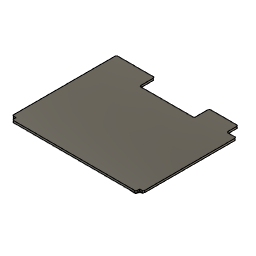
HexDeck_Printed_v0.1 (Autodesk Fusion 360 design; units mm, degrees)
Autodesk Fusion 360 part; units mm, degrees
(part 1 of 2)
sketch "Sketch1" plane through (0, 0, 86) normal (0, 0, 1) x (-1, 0, 0)
  line L0 (-104.5, -11) -> (-104.5, -155)
  arc A0 (-104.5, -155) -> (-102.5, -157) centre (-102.5, -155) ccw
  line L1 (-102.5, -157) -> (-91.5, -157)
  arc A1 (-89.5, -159) -> (-91.5, -157) centre (-91.5, -159) ccw
  line L2 (-89.5, -159) -> (-89.5, -173)
  arc A2 (-89.5, -173) -> (-87.5, -175) centre (-87.5, -173) ccw
  line L3 (-87.5, -175) -> (-45.5, -175)
  arc A3 (-45.5, -175) -> (-43.5, -173) centre (-45.5, -173) ccw
  line L4 (-43.5, -173) -> (-43.5, -153)
  arc A4 (-41.5, -151) -> (-43.5, -153) centre (-41.5, -153) ccw
  line L5 (-41.5, -151) -> (41.5, -151)
  arc A5 (43.5, -153) -> (41.5, -151) centre (41.5, -153) ccw
  line L6 (43.5, -153) -> (43.5, -173)
  arc A6 (43.5, -173) -> (45.5, -175) centre (45.5, -173) ccw
  arc A7 (98.5, -8.5) -> (99, -9) centre (99, -8.5) ccw
  line L7 (98.5, -8.5) -> (98.5, -5)
  arc A8 (98.5, -5) -> (96.5, -3) centre (96.5, -5) ccw
  line L8 (96.5, -3) -> (-96.5, -3)
  arc A9 (-96.5, -3) -> (-98.5, -5) centre (-96.5, -5) ccw
  line L9 (-98.5, -5) -> (-98.5, -8.5)
  arc A10 (-99, -9) -> (-98.5, -8.5) centre (-99, -8.5) ccw
  line L10 (-99, -9) -> (-102.5, -9)
  arc A11 (-102.5, -9) -> (-104.5, -11) centre (-102.5, -11) ccw
  circle A12 centre (-6, -134.5) radius 1.75
  circle A13 centre (-91, -12) radius 1.75
  circle A14 centre (85.1504, -110.8568) radius 1.7
  circle A15 centre (20.415, -94.6658) radius 1.7
  circle A16 centre (57.915, -46.1658) radius 1.7
  circle A17 centre (20.415, -32.4658) radius 1.7
  circle A18 centre (55.415, -14.2658) radius 1.7
  circle A19 centre (-91, -12) radius 1.75
  line L11 (100, -13.5) -> (99, -13.5)
  arc A20 (94, -8.5) -> (99, -13.5) centre (99, -8.5) ccw
  line L12 (94, -8.5) -> (94, -7.5)
  line L13 (94, -7.5) -> (-94, -7.5)
  line L14 (-94, -7.5) -> (-94, -8.5)
  arc A21 (-99, -13.5) -> (-94, -8.5) centre (-99, -8.5) ccw
  line L15 (-99, -13.5) -> (-100, -13.5)
  line L16 (-100, -13.5) -> (-100, -152.5)
  line L17 (-100, -152.5) -> (-91.5, -152.5)
  arc A22 (-85, -159) -> (-91.5, -152.5) centre (-91.5, -159) ccw
  line L18 (-85, -159) -> (-85, -170.5)
  line L19 (-85, -170.5) -> (-48, -170.5)
  line L20 (-48, -170.5) -> (-48, -153)
  arc A23 (-41.5, -146.5) -> (-48, -153) centre (-41.5, -153) ccw
  line L21 (-41.5, -146.5) -> (41.5, -146.5)
  arc A24 (48, -153) -> (41.5, -146.5) centre (41.5, -153) ccw
  line L22 (48, -153) -> (48, -170.5)
  line L23 (48, -170.5) -> (100, -170.5)
  line L24 (100, -170.5) -> (100, -13.5)
  line L25 (-92.8571, -14.0158) -> (-87.2143, -10.7579)
  line L26 (-87.2143, -10.7579) -> (-87.2143, -7.5)
  line L27 (-95.7822, -12.327) -> (-92.8571, -14.0158)
  line L28 (-100, -26.3876) -> (-94.3571, -23.1297)
  line L29 (-94.3571, -23.1297) -> (-94.3572, -16.6139)
  line L30 (-94.3572, -16.6139) -> (-99.7505, -13.5)
  line L31 (0, 0) -> (0, -167.5443) construction
  line L32 (100, -55) -> (-100, -55) construction
  line L33 (-72.9286, -10.7579) -> (-72.9286, -7.5)
  line L34 (-84.2143, -7.5) -> (-84.2143, -10.7579)
  line L35 (-78.5714, -14.0158) -> (-72.9286, -10.7579)
  line L36 (-84.2143, -10.7579) -> (-78.5714, -14.0158)
  line L37 (-91.3571, -16.6139) -> (-91.3571, -23.1297)
  line L38 (-91.3571, -23.1297) -> (-85.7143, -26.3876)
  line L39 (-85.7143, -26.3876) -> (-80.0714, -23.1297)
  line L40 (-80.0714, -23.1297) -> (-80.0714, -16.6139)
  line L41 (-85.7143, -13.356) -> (-91.3571, -16.6139)
  line L42 (-80.0714, -16.6139) -> (-85.7143, -13.356)
  line L43 (-58.6429, -10.7579) -> (-58.6429, -7.5)
  line L44 (-69.9286, -7.5) -> (-69.9286, -10.7579)
  line L45 (-64.2857, -14.0158) -> (-58.6429, -10.7579)
  line L46 (-69.9286, -10.7579) -> (-64.2857, -14.0158)
  line L47 (-77.0714, -16.6139) -> (-77.0714, -23.1297)
  line L48 (-77.0714, -23.1297) -> (-71.4286, -26.3876)
  line L49 (-71.4286, -26.3876) -> (-65.7857, -23.1297)
  line L50 (-65.7857, -23.1297) -> (-65.7857, -16.6139)
  line L51 (-71.4286, -13.356) -> (-77.0714, -16.6139)
  line L52 (-65.7857, -16.6139) -> (-71.4286, -13.356)
  line L53 (-44.3572, -10.7579) -> (-44.3572, -7.5)
  line L54 (-55.6429, -7.5) -> (-55.6429, -10.7579)
  line L55 (-50, -14.0158) -> (-44.3572, -10.7579)
  line L56 (-55.6429, -10.7579) -> (-50, -14.0158)
  line L57 (-62.7857, -16.6139) -> (-62.7857, -23.1297)
  line L58 (-62.7857, -23.1297) -> (-57.1429, -26.3876)
  line L59 (-57.1429, -26.3876) -> (-51.5, -23.1297)
  line L60 (-51.5, -23.1297) -> (-51.5, -16.6139)
  line L61 (-57.1429, -13.356) -> (-62.7857, -16.6139)
  line L62 (-51.5, -16.6139) -> (-57.1429, -13.356)
  line L63 (-30.0714, -10.7579) -> (-30.0714, -7.5)
  line L64 (-41.3571, -7.5) -> (-41.3571, -10.7579)
  line L65 (-35.7143, -14.0158) -> (-30.0714, -10.7579)
  line L66 (-41.3571, -10.7579) -> (-35.7143, -14.0158)
  line L67 (-48.5, -16.6139) -> (-48.5, -23.1297)
  line L68 (-48.5, -23.1297) -> (-42.8571, -26.3876)
  line L69 (-42.8571, -26.3876) -> (-37.2143, -23.1297)
  line L70 (-37.2143, -23.1297) -> (-37.2143, -16.6139)
  line L71 (-42.8571, -13.356) -> (-48.5, -16.6139)
  line L72 (-37.2143, -16.6139) -> (-42.8571, -13.356)
  line L73 (-15.7857, -10.7579) -> (-15.7857, -7.5)
  line L74 (-27.0714, -7.5) -> (-27.0714, -10.7579)
  line L75 (-21.4286, -14.0158) -> (-15.7857, -10.7579)
  line L76 (-27.0714, -10.7579) -> (-21.4286, -14.0158)
  line L77 (-34.2143, -16.6139) -> (-34.2143, -23.1297)
  line L78 (-34.2143, -23.1297) -> (-28.5714, -26.3876)
  line L79 (-28.5714, -26.3876) -> (-22.9286, -23.1297)
  line L80 (-22.9286, -23.1297) -> (-22.9286, -16.6139)
  line L81 (-28.5714, -13.356) -> (-34.2143, -16.6139)
  line L82 (-22.9286, -16.6139) -> (-28.5714, -13.356)
  line L83 (-1.5, -10.7579) -> (-1.5, -7.5)
  line L84 (-12.7857, -7.5) -> (-12.7857, -10.7579)
  line L85 (-7.1429, -14.0158) -> (-1.5, -10.7579)
  line L86 (-12.7857, -10.7579) -> (-7.1429, -14.0158)
  line L87 (-19.9286, -16.6139) -> (-19.9286, -23.1297)
  line L88 (-19.9286, -23.1297) -> (-14.2857, -26.3876)
  line L89 (-14.2857, -26.3876) -> (-8.6429, -23.1297)
  line L90 (-8.6429, -23.1297) -> (-8.6429, -16.6139)
  line L91 (-14.2857, -13.356) -> (-19.9286, -16.6139)
  line L92 (-8.6429, -16.6139) -> (-14.2857, -13.356)
  line L93 (12.7857, -10.7579) -> (12.7857, -7.5)
  line L94 (1.5, -4.2421) -> (1.5, -10.7579)
  line L95 (7.1428, -14.0158) -> (12.7857, -10.7579)
  line L96 (1.5, -10.7579) -> (7.1428, -14.0158)
  line L97 (-5.6429, -16.6139) -> (-5.6429, -23.1297)
  line L98 (-5.6429, -23.1297) -> (0, -26.3876)
  line L99 (0, -26.3876) -> (5.6428, -23.1297)
  line L100 (5.6428, -23.1297) -> (5.6428, -16.6139)
  line L101 (0, -13.356) -> (-5.6429, -16.6139)
  line L102 (5.6428, -16.6139) -> (0, -13.356)
  line L103 (27.0714, -10.7579) -> (27.0714, -7.5)
  line L104 (15.7857, -7.5) -> (15.7857, -10.7579)
  line L105 (21.4286, -14.0158) -> (27.0714, -10.7579)
  line L106 (15.7857, -10.7579) -> (21.4286, -14.0158)
  line L107 (8.6429, -16.6139) -> (8.6429, -23.1301)
  line L108 (8.6429, -23.1301) -> (14.2857, -26.388)
  line L109 (19.9286, -23.1301) -> (19.9286, -16.6139)
  line L110 (14.2857, -13.356) -> (8.6429, -16.6139)
  line L111 (19.9286, -16.6139) -> (14.2857, -13.356)
  line L112 (41.3571, -10.7579) -> (41.3571, -7.5)
  line L113 (30.0714, -7.5) -> (30.0714, -10.7579)
  line L114 (35.7143, -14.0158) -> (41.3571, -10.7579)
  line L115 (30.0714, -10.7579) -> (35.7143, -14.0158)
  line L116 (22.9282, -16.6141) -> (22.9282, -23.1299)
  line L117 (28.571, -26.3878) -> (34.2143, -23.1297)
  line L118 (34.2143, -23.1297) -> (34.2143, -16.6139)
  line L119 (28.5714, -13.356) -> (22.9282, -16.6141)
  line L120 (34.2143, -16.6139) -> (28.5714, -13.356)
  line L121 (55.6423, -10.7579) -> (55.6423, -7.5)
  line L122 (44.3571, -7.5) -> (44.3571, -10.7574)
  line L123 (44.3571, -10.7574) -> (50, -14.0153)
  line L124 (37.2143, -16.6139) -> (37.2143, -23.1297)
  line L125 (37.2143, -23.1297) -> (42.8571, -26.3876)
  line L126 (42.8571, -26.3876) -> (48.4995, -23.1299)
  line L127 (42.8569, -13.3561) -> (37.2143, -16.6139)
  line L128 (48.4997, -16.6141) -> (42.8569, -13.3561)
  line L129 (69.9286, -10.7576) -> (69.9286, -7.5)
  line L130 (58.6438, -7.5) -> (58.6438, -10.7579)
  line L131 (64.2857, -14.0155) -> (69.9286, -10.7576)
  line L132 (51.5, -16.6139) -> (51.5, -23.1297)
  line L133 (51.5, -23.1297) -> (57.1429, -26.3876)
  line L134 (57.1429, -26.3876) -> (62.7857, -23.1297)
  line L135 (62.7857, -23.1297) -> (62.7857, -16.6139)
  line L136 (57.1429, -13.356) -> (51.5, -16.6139)
  line L137 (62.7857, -16.6139) -> (57.1429, -13.356)
  line L138 (84.2143, -10.7579) -> (84.2143, -7.5)
  line L139 (72.9286, -7.5) -> (72.9286, -10.7579)
  line L140 (78.5714, -14.0158) -> (84.2143, -10.7579)
  line L141 (72.9286, -10.7579) -> (78.5714, -14.0158)
  line L142 (65.786, -23.1295) -> (71.4289, -26.3874)
  line L143 (71.4289, -26.3874) -> (77.0714, -23.1297)
  line L144 (77.0714, -23.1297) -> (77.0714, -16.6139)
  line L145 (71.4286, -13.356) -> (65.7862, -16.6136)
  line L146 (77.0714, -16.6139) -> (71.4286, -13.356)
  line L147 (87.2143, -7.5) -> (87.2143, -10.7579)
  line L148 (92.8571, -14.0158) -> (95.7822, -12.327)
  line L149 (87.2143, -10.7579) -> (92.8571, -14.0158)
  line L150 (80.0714, -16.6139) -> (80.0714, -23.1297)
  line L151 (80.0714, -23.1297) -> (85.7143, -26.3876)
  line L152 (85.7143, -26.3876) -> (91.3571, -23.1297)
  line L153 (91.3571, -23.1297) -> (91.3571, -16.6139)
  line L154 (85.7143, -13.356) -> (80.0714, -16.6139)
  line L155 (91.3571, -16.6139) -> (85.7143, -13.356)
  line L156 (94.3571, -16.6139) -> (94.3571, -23.1297)
  line L157 (94.3571, -23.1297) -> (100, -26.3876)
  line L158 (99.7505, -13.5) -> (94.3571, -16.6139)
  line L159 (-87.2143, -35.5019) -> (-87.2143, -28.9861)
  line L160 (-87.2143, -28.9861) -> (-92.8572, -25.7282)
  line L161 (-92.8572, -25.7282) -> (-98.5, -28.9861)
  line L162 (-98.5, -28.9861) -> (-98.5, -35.5019)
  line L163 (-92.8571, -38.7598) -> (-87.2143, -35.5019)
  line L164 (-98.5, -35.5019) -> (-92.8571, -38.7598)
  line L165 (-100, -51.1316) -> (-94.3571, -47.8737)
  line L166 (-94.3571, -47.8737) -> (-94.3572, -41.3579)
  line L167 (-94.3572, -41.3579) -> (-100, -38.1)
  line L168 (-72.9286, -35.5019) -> (-72.9286, -28.9861)
  line L169 (-72.9286, -28.9861) -> (-78.5714, -25.7282)
  line L170 (-78.5714, -25.7282) -> (-84.2143, -28.9861)
  line L171 (-84.2143, -28.9861) -> (-84.2143, -35.5019)
  line L172 (-78.5714, -38.7598) -> (-72.9286, -35.5019)
  line L173 (-84.2143, -35.5019) -> (-78.5714, -38.7598)
  line L174 (-91.3571, -41.3579) -> (-91.3571, -47.8737)
  line L175 (-91.3571, -47.8737) -> (-85.7143, -51.1316)
  line L176 (-85.7143, -51.1316) -> (-80.0714, -47.8737)
  line L177 (-80.0714, -47.8737) -> (-80.0714, -41.3579)
  line L178 (-85.7143, -38.1) -> (-91.3571, -41.3579)
  line L179 (-80.0714, -41.3579) -> (-85.7143, -38.1)
  line L180 (-58.6429, -35.5019) -> (-58.6429, -28.9861)
  line L181 (-58.6429, -28.9861) -> (-64.2857, -25.7282)
  line L182 (-64.2857, -25.7282) -> (-69.9286, -28.9861)
  line L183 (-69.9286, -28.9861) -> (-69.9286, -35.5019)
  line L184 (-64.2857, -38.7598) -> (-58.6429, -35.5019)
  line L185 (-69.9286, -35.5019) -> (-64.2857, -38.7598)
  line L186 (-77.0714, -41.3579) -> (-77.0714, -47.8737)
  line L187 (-77.0714, -47.8737) -> (-71.4286, -51.1316)
  line L188 (-71.4286, -51.1316) -> (-65.7857, -47.8737)
  line L189 (-65.7857, -47.8737) -> (-65.7857, -41.3579)
  line L190 (-71.4286, -38.1) -> (-77.0714, -41.3579)
  line L191 (-65.7857, -41.3579) -> (-71.4286, -38.1)
  line L192 (-44.3572, -35.5019) -> (-44.3572, -28.9861)
  line L193 (-44.3572, -28.9861) -> (-50, -25.7282)
  line L194 (-50, -25.7282) -> (-55.6429, -28.9861)
  line L195 (-55.6429, -28.9861) -> (-55.6429, -35.5019)
  line L196 (-50, -38.7598) -> (-44.3572, -35.5019)
  line L197 (-55.6429, -35.5019) -> (-50, -38.7598)
  line L198 (-62.7857, -41.3579) -> (-62.7857, -47.8737)
  line L199 (-62.7857, -47.8737) -> (-57.1429, -51.1316)
  line L200 (-57.1429, -51.1316) -> (-51.5, -47.8737)
  line L201 (-51.5, -47.8737) -> (-51.5, -41.3579)
  line L202 (-57.1429, -38.1) -> (-62.7857, -41.3579)
  line L203 (-51.5, -41.3579) -> (-57.1429, -38.1)
  line L204 (-30.0714, -35.5019) -> (-30.0714, -28.9861)
  line L205 (-30.0714, -28.9861) -> (-35.7143, -25.7282)
  line L206 (-35.7143, -25.7282) -> (-41.3571, -28.9861)
  line L207 (-41.3571, -28.9861) -> (-41.3571, -35.5019)
  line L208 (-35.7143, -38.7598) -> (-30.0714, -35.5019)
  line L209 (-41.3571, -35.5019) -> (-35.7143, -38.7598)
  line L210 (-48.5, -41.3579) -> (-48.5, -47.8737)
  line L211 (-48.5, -47.8737) -> (-42.8571, -51.1316)
  line L212 (-42.8571, -51.1316) -> (-37.2143, -47.8737)
  line L213 (-37.2143, -47.8737) -> (-37.2143, -41.3579)
  line L214 (-42.8571, -38.1) -> (-48.5, -41.3579)
  line L215 (-37.2143, -41.3579) -> (-42.8571, -38.1)
  line L216 (-15.7857, -35.5019) -> (-15.7857, -28.9861)
  line L217 (-15.7857, -28.9861) -> (-21.4286, -25.7282)
  line L218 (-21.4286, -25.7282) -> (-27.0714, -28.9861)
  line L219 (-27.0714, -28.9861) -> (-27.0714, -35.5019)
  line L220 (-21.4286, -38.7598) -> (-15.7857, -35.5019)
  line L221 (-27.0714, -35.5019) -> (-21.4286, -38.7598)
  line L222 (-34.2143, -41.3579) -> (-34.2143, -47.8737)
  line L223 (-34.2143, -47.8737) -> (-28.5714, -51.1316)
  line L224 (-28.5714, -51.1316) -> (-22.9286, -47.8737)
  line L225 (-22.9286, -47.8737) -> (-22.9286, -41.3579)
  line L226 (-28.5714, -38.1) -> (-34.2143, -41.3579)
  line L227 (-22.9286, -41.3579) -> (-28.5714, -38.1)
  line L228 (-1.5, -35.5019) -> (-1.5, -28.9861)
  line L229 (-1.5, -28.9861) -> (-7.1429, -25.7282)
  line L230 (-7.1429, -25.7282) -> (-12.7857, -28.9861)
  line L231 (-12.7857, -28.9861) -> (-12.7857, -35.5019)
  line L232 (-7.1429, -38.7598) -> (-1.5, -35.5019)
  line L233 (-12.7857, -35.5019) -> (-7.1429, -38.7598)
  line L234 (-19.9286, -41.3579) -> (-19.9286, -47.8737)
  line L235 (-19.9286, -47.8737) -> (-14.2857, -51.1316)
  line L236 (-14.2857, -51.1316) -> (-8.6429, -47.8737)
  line L237 (-8.6429, -47.8737) -> (-8.6429, -41.3579)
  line L238 (-14.2857, -38.1) -> (-19.9286, -41.3579)
  line L239 (-8.6429, -41.3579) -> (-14.2857, -38.1)
  line L240 (12.7857, -28.9861) -> (7.1428, -25.7282)
  line L241 (7.1428, -25.7282) -> (1.5, -28.9861)
  line L242 (1.5, -28.9861) -> (1.5, -35.5019)
  line L243 (7.1429, -38.7598) -> (12.7857, -35.5019)
  line L244 (1.5, -35.5019) -> (7.1429, -38.7598)
  line L245 (-5.6429, -41.3579) -> (-5.6429, -47.8737)
  line L246 (-5.6429, -47.8737) -> (0, -51.1316)
  line L247 (0, -51.1316) -> (5.6428, -47.8737)
  line L248 (5.6428, -47.8737) -> (5.6428, -41.3579)
  line L249 (0, -38.1) -> (-5.6429, -41.3579)
  line L250 (5.6428, -41.3579) -> (0, -38.1)
  line L251 (27.0714, -35.5019) -> (27.0714, -28.9861)
  line L252 (27.0714, -28.9861) -> (21.4286, -25.7282)
  line L253 (21.4286, -25.7282) -> (15.7857, -28.9861)
  line L254 (15.7857, -28.9861) -> (15.7857, -35.5019)
  line L255 (21.4286, -38.7598) -> (27.0714, -35.5019)
  line L256 (15.7857, -35.5019) -> (21.4286, -38.7598)
  line L257 (8.6429, -41.3579) -> (8.6429, -47.8737)
  line L258 (8.6429, -47.8737) -> (14.2857, -51.1316)
  line L259 (14.2857, -51.1316) -> (19.9286, -47.8737)
  line L260 (19.9286, -47.8737) -> (19.9286, -41.3579)
  line L261 (14.2857, -38.1) -> (8.6429, -41.3579)
  line L262 (41.3571, -35.5019) -> (41.3571, -28.9861)
  line L263 (41.3571, -28.9861) -> (35.7143, -25.7282)
  line L264 (35.7143, -25.7282) -> (30.0714, -28.9861)
  line L265 (35.7143, -38.7598) -> (41.3571, -35.5019)
  line L266 (30.0714, -35.5019) -> (35.7143, -38.7598)
  line L267 (22.9286, -41.3579) -> (22.9286, -47.8737)
  line L268 (22.9286, -47.8737) -> (28.5714, -51.1316)
  line L269 (28.5714, -51.1316) -> (34.2143, -47.8737)
  line L270 (34.2143, -47.8737) -> (34.2143, -41.3579)
  line L271 (34.2143, -41.3579) -> (28.5714, -38.1)
  line L272 (55.6428, -35.5019) -> (55.6428, -28.9861)
  line L273 (50, -25.7281) -> (44.3571, -28.986)
  line L274 (44.3571, -28.986) -> (44.3571, -35.5019)
  line L275 (44.3571, -35.5019) -> (50, -38.7598)
  line L276 (37.2143, -41.3579) -> (37.2143, -47.8737)
  line L277 (37.2143, -47.8737) -> (42.8571, -51.1316)
  line L278 (42.8571, -51.1316) -> (48.5, -47.8737)
  line L279 (42.8571, -38.1) -> (37.2143, -41.3579)
  line L280 (48.5, -41.3579) -> (42.8571, -38.1)
  line L281 (69.9287, -35.5019) -> (69.9286, -28.9861)
  line L282 (69.9286, -28.9861) -> (64.2858, -25.7282)
  line L283 (58.6428, -28.986) -> (58.6428, -35.5018)
  line L284 (64.2858, -38.7598) -> (69.9287, -35.5019)
  line L285 (51.5, -41.3579) -> (51.5, -47.8737)
  line L286 (51.5, -47.8737) -> (57.1429, -51.1316)
  line L287 (57.1429, -51.1316) -> (62.7857, -47.8737)
  line L288 (62.7857, -47.8737) -> (62.7857, -41.3579)
  line L289 (57.1429, -38.1) -> (51.5, -41.3579)
  line L290 (62.7857, -41.3579) -> (57.1429, -38.1)
  line L291 (84.2143, -35.5019) -> (84.2143, -28.9861)
  line L292 (84.2143, -28.9861) -> (78.5714, -25.7282)
  line L293 (78.5714, -25.7282) -> (72.9286, -28.9861)
  line L294 (72.9286, -28.9861) -> (72.9286, -35.5019)
  line L295 (78.5714, -38.7598) -> (84.2143, -35.5019)
  line L296 (72.9286, -35.5019) -> (78.5714, -38.7598)
  line L297 (65.7857, -47.8737) -> (71.4286, -51.1316)
  line L298 (71.4286, -51.1316) -> (77.0714, -47.8737)
  line L299 (77.0714, -47.8737) -> (77.0714, -41.3579)
  line L300 (71.4286, -38.1) -> (65.7857, -41.3579)
  line L301 (77.0714, -41.3579) -> (71.4286, -38.1)
  line L302 (98.5, -35.5019) -> (98.5, -28.9861)
  line L303 (98.5, -28.9861) -> (92.8571, -25.7282)
  line L304 (92.8571, -25.7282) -> (87.2143, -28.9861)
  line L305 (87.2143, -28.9861) -> (87.2143, -35.5019)
  line L306 (92.8571, -38.7598) -> (98.5, -35.5019)
  line L307 (87.2143, -35.5019) -> (92.8571, -38.7598)
  line L308 (80.0714, -41.3579) -> (80.0714, -47.8737)
  line L309 (80.0714, -47.8737) -> (85.7143, -51.1316)
  line L310 (85.7143, -51.1316) -> (91.3571, -47.8737)
  line L311 (91.3571, -47.8737) -> (91.3571, -41.3579)
  line L312 (85.7143, -38.1) -> (80.0714, -41.3579)
  line L313 (91.3571, -41.3579) -> (85.7143, -38.1)
  line L314 (94.3571, -41.3579) -> (94.3571, -47.8737)
  line L315 (94.3571, -47.8737) -> (100, -51.1316)
  line L316 (100, -38.1) -> (94.3571, -41.3579)
  line L317 (-87.2143, -60.2459) -> (-87.2143, -53.7301)
  line L318 (-87.2143, -53.7301) -> (-92.8572, -50.4722)
  line L319 (-92.8572, -50.4722) -> (-98.5, -53.7301)
  line L320 (-98.5, -53.7301) -> (-98.5, -60.2459)
  line L321 (-92.8571, -63.5038) -> (-87.2143, -60.2459)
  line L322 (-98.5, -60.2459) -> (-92.8571, -63.5038)
  line L323 (-100, -75.8756) -> (-94.3571, -72.6177)
  line L324 (-94.3571, -72.6177) -> (-94.3572, -66.1019)
  line L325 (-94.3572, -66.1019) -> (-100, -62.844)
  line L326 (-72.9286, -60.2459) -> (-72.9286, -53.7301)
  line L327 (-72.9286, -53.7301) -> (-78.5714, -50.4722)
  line L328 (-78.5714, -50.4722) -> (-84.2143, -53.7301)
  line L329 (-84.2143, -53.7301) -> (-84.2143, -60.2459)
  line L330 (-78.5714, -63.5038) -> (-72.9286, -60.2459)
  line L331 (-84.2143, -60.2459) -> (-78.5714, -63.5038)
  line L332 (-91.3571, -66.1019) -> (-91.3571, -72.6177)
  line L333 (-91.3571, -72.6177) -> (-85.7143, -75.8756)
  line L334 (-85.7143, -75.8756) -> (-80.0714, -72.6177)
  line L335 (-80.0714, -72.6177) -> (-80.0714, -66.1019)
  line L336 (-85.7143, -62.844) -> (-91.3571, -66.1019)
  line L337 (-80.0714, -66.1019) -> (-85.7143, -62.844)
  line L338 (-58.6429, -60.2459) -> (-58.6429, -53.7301)
  line L339 (-58.6429, -53.7301) -> (-64.2857, -50.4722)
  line L340 (-64.2857, -50.4722) -> (-69.9286, -53.7301)
  line L341 (-69.9286, -53.7301) -> (-69.9286, -60.2459)
  line L342 (-64.2857, -63.5038) -> (-58.6429, -60.2459)
  line L343 (-69.9286, -60.2459) -> (-64.2857, -63.5038)
  line L344 (-77.0714, -66.1019) -> (-77.0714, -72.6177)
  line L345 (-77.0714, -72.6177) -> (-71.4286, -75.8756)
  line L346 (-71.4286, -75.8756) -> (-65.7857, -72.6177)
  line L347 (-65.7857, -72.6177) -> (-65.7857, -66.1019)
  line L348 (-71.4286, -62.844) -> (-77.0714, -66.1019)
  line L349 (-65.7857, -66.1019) -> (-71.4286, -62.844)
  line L350 (-44.3572, -60.2459) -> (-44.3572, -53.7301)
  line L351 (-44.3572, -53.7301) -> (-50, -50.4722)
  line L352 (-50, -50.4722) -> (-55.6429, -53.7301)
  line L353 (-55.6429, -53.7301) -> (-55.6429, -60.2459)
  line L354 (-50, -63.5038) -> (-44.3572, -60.2459)
  line L355 (-55.6429, -60.2459) -> (-50, -63.5038)
  line L356 (-62.7857, -66.1019) -> (-62.7857, -72.6177)
  line L357 (-62.7857, -72.6177) -> (-57.1429, -75.8756)
  line L358 (-57.1429, -75.8756) -> (-51.5, -72.6177)
  line L359 (-51.5, -72.6177) -> (-51.5, -66.1019)
  line L360 (-57.1429, -62.844) -> (-62.7857, -66.1019)
  line L361 (-51.5, -66.1019) -> (-57.1429, -62.844)
  line L362 (-30.0714, -60.2459) -> (-30.0714, -53.7301)
  line L363 (-30.0714, -53.7301) -> (-35.7143, -50.4722)
  line L364 (-35.7143, -50.4722) -> (-41.3571, -53.7301)
  line L365 (-41.3571, -53.7301) -> (-41.3571, -60.2459)
  line L366 (-35.7143, -63.5038) -> (-30.0714, -60.2459)
  line L367 (-41.3571, -60.2459) -> (-35.7143, -63.5038)
  line L368 (-48.5, -66.1019) -> (-48.5, -72.6177)
  line L369 (-48.5, -72.6177) -> (-42.8571, -75.8756)
  line L370 (-42.8571, -75.8756) -> (-37.2143, -72.6177)
  line L371 (-37.2143, -72.6177) -> (-37.2143, -66.1019)
  line L372 (-42.8571, -62.844) -> (-48.5, -66.1019)
  line L373 (-37.2143, -66.1019) -> (-42.8571, -62.844)
  line L374 (-15.7857, -60.2459) -> (-15.7857, -53.7301)
  line L375 (-15.7857, -53.7301) -> (-21.4286, -50.4722)
  line L376 (-21.4286, -50.4722) -> (-27.0714, -53.7301)
  line L377 (-27.0714, -53.7301) -> (-27.0714, -60.2459)
  line L378 (-21.4286, -63.5038) -> (-15.7857, -60.2459)
  line L379 (-27.0714, -60.2459) -> (-21.4286, -63.5038)
  line L380 (-34.2143, -66.1019) -> (-34.2143, -72.6177)
  line L381 (-34.2143, -72.6177) -> (-28.5714, -75.8756)
  line L382 (-28.5714, -75.8756) -> (-22.9286, -72.6177)
  line L383 (-22.9286, -72.6177) -> (-22.9286, -66.1019)
  line L384 (-28.5714, -62.844) -> (-34.2143, -66.1019)
  line L385 (-22.9286, -66.1019) -> (-28.5714, -62.844)
  line L386 (-1.5, -60.2459) -> (-1.5, -53.7301)
  line L387 (-1.5, -53.7301) -> (-7.1429, -50.4722)
  line L388 (-7.1429, -50.4722) -> (-12.7857, -53.7301)
  line L389 (-12.7857, -53.7301) -> (-12.7857, -60.2459)
  line L390 (-7.1429, -63.5038) -> (-1.5, -60.2459)
  line L391 (-12.7857, -60.2459) -> (-7.1429, -63.5038)
  line L392 (-19.9286, -66.1019) -> (-19.9286, -72.6177)
  line L393 (-19.9286, -72.6177) -> (-14.2857, -75.8756)
  line L394 (-14.2857, -75.8756) -> (-8.6429, -72.6177)
  line L395 (-8.6429, -72.6177) -> (-8.6429, -66.1019)
  line L396 (-14.2857, -62.844) -> (-19.9286, -66.1019)
  line L397 (-8.6429, -66.1019) -> (-14.2857, -62.844)
  line L398 (12.7857, -60.2459) -> (12.7857, -53.7301)
  line L399 (12.7857, -53.7301) -> (7.1428, -50.4722)
  line L400 (7.1428, -50.4722) -> (1.5, -53.7301)
  line L401 (1.5, -53.7301) -> (1.5, -60.2459)
  line L402 (7.1428, -63.5038) -> (12.7857, -60.2459)
  line L403 (1.5, -60.2459) -> (7.1428, -63.5038)
  line L404 (-5.6429, -66.1019) -> (-5.6429, -72.6177)
  line L405 (-5.6429, -72.6177) -> (0, -75.8756)
  line L406 (0, -75.8756) -> (5.6428, -72.6177)
  line L407 (5.6428, -72.6177) -> (5.6428, -66.1019)
  line L408 (0, -62.844) -> (-5.6429, -66.1019)
  line L409 (5.6428, -66.1019) -> (0, -62.844)
  line L410 (27.0714, -60.2459) -> (27.0714, -53.7301)
  line L411 (27.0714, -53.7301) -> (21.4286, -50.4722)
  line L412 (21.4286, -50.4722) -> (15.7857, -53.7301)
  line L413 (15.7857, -53.7301) -> (15.7857, -60.2459)
  line L414 (21.4286, -63.5038) -> (27.0714, -60.2459)
  line L415 (15.7857, -60.2459) -> (21.4286, -63.5038)
  line L416 (8.6429, -66.1019) -> (8.6429, -72.6177)
  line L417 (8.6429, -72.6177) -> (14.2857, -75.8756)
  line L418 (14.2857, -75.8756) -> (19.9286, -72.6177)
  line L419 (19.9286, -72.6177) -> (19.9286, -66.1019)
  line L420 (14.2857, -62.844) -> (8.6429, -66.1019)
  line L421 (19.9286, -66.1019) -> (14.2857, -62.844)
  line L422 (41.3571, -60.2459) -> (41.3571, -53.7301)
  line L423 (41.3571, -53.7301) -> (35.7143, -50.4722)
  line L424 (35.7143, -50.4722) -> (30.0714, -53.7301)
  line L425 (30.0714, -53.7301) -> (30.0714, -60.2459)
  line L426 (35.7143, -63.5038) -> (41.3571, -60.2459)
  line L427 (30.0714, -60.2459) -> (35.7143, -63.5038)
  line L428 (22.9286, -66.1019) -> (22.9286, -72.6177)
  line L429 (22.9286, -72.6177) -> (28.5714, -75.8756)
  line L430 (28.5714, -75.8756) -> (34.2143, -72.6177)
  line L431 (34.2143, -72.6177) -> (34.2143, -66.1019)
  line L432 (28.5714, -62.844) -> (22.9286, -66.1019)
  line L433 (34.2143, -66.1019) -> (28.5714, -62.844)
  line L434 (55.6432, -60.2457) -> (55.6432, -53.7299)
  line L435 (50.0004, -50.472) -> (44.3571, -53.7301)
  line L436 (44.3571, -53.7301) -> (44.3571, -60.2459)
  line L437 (50, -63.5038) -> (55.6432, -60.2457)
  line L438 (44.3571, -60.2459) -> (50, -63.5038)
  line L439 (37.2143, -66.1019) -> (37.2143, -72.6177)
  line L440 (37.2143, -72.6177) -> (42.8571, -75.8756)
  line L441 (42.8571, -75.8756) -> (48.5, -72.6177)
  line L442 (48.5, -72.6177) -> (48.5, -66.1019)
  line L443 (42.8571, -62.844) -> (37.2143, -66.1019)
  line L444 (48.5, -66.1019) -> (42.8571, -62.844)
  line L445 (69.9286, -60.2459) -> (69.9286, -53.7297)
  line L446 (69.9286, -53.7297) -> (64.2857, -50.4718)
  line L447 (58.6429, -53.7297) -> (58.6429, -60.2459)
  line L448 (64.2857, -63.5038) -> (69.9286, -60.2459)
  line L449 (58.6429, -60.2459) -> (64.2857, -63.5038)
  line L450 (51.5, -66.1019) -> (51.5, -72.6177)
  line L451 (51.5, -72.6177) -> (57.1429, -75.8756)
  line L452 (57.1429, -75.8756) -> (62.7857, -72.6177)
  line L453 (62.7857, -72.6177) -> (62.7857, -66.1019)
  line L454 (57.1429, -62.844) -> (51.5, -66.1019)
  line L455 (62.7857, -66.1019) -> (57.1429, -62.844)
  line L456 (84.2143, -60.2459) -> (84.2143, -53.7301)
  line L457 (84.2143, -53.7301) -> (78.5714, -50.4722)
  line L458 (78.5714, -50.4722) -> (72.9286, -53.7301)
  line L459 (72.9286, -53.7301) -> (72.9286, -60.2459)
  line L460 (78.5714, -63.5038) -> (84.2143, -60.2459)
  line L461 (72.9286, -60.2459) -> (78.5714, -63.5038)
  line L462 (65.7857, -66.1019) -> (65.7857, -72.6177)
  line L463 (65.7857, -72.6177) -> (71.4286, -75.8756)
  line L464 (71.4286, -75.8756) -> (77.0714, -72.6177)
  line L465 (77.0714, -72.6177) -> (77.0714, -66.1019)
  line L466 (71.4286, -62.844) -> (65.7857, -66.1019)
  line L467 (77.0714, -66.1019) -> (71.4286, -62.844)
  line L468 (98.5, -60.2459) -> (98.5, -53.7301)
  line L469 (98.5, -53.7301) -> (92.8571, -50.4722)
  line L470 (92.8571, -50.4722) -> (87.2143, -53.7301)
  line L471 (87.2143, -53.7301) -> (87.2143, -60.2459)
  line L472 (92.8571, -63.5038) -> (98.5, -60.2459)
  line L473 (87.2143, -60.2459) -> (92.8571, -63.5038)
  line L474 (80.0714, -66.1019) -> (80.0714, -72.6177)
  line L475 (80.0714, -72.6177) -> (85.7143, -75.8756)
  line L476 (85.7143, -75.8756) -> (91.3571, -72.6177)
  line L477 (91.3571, -72.6177) -> (91.3571, -66.1019)
  line L478 (85.7143, -62.844) -> (80.0714, -66.1019)
  line L479 (91.3571, -66.1019) -> (85.7143, -62.844)
  line L480 (94.3571, -66.1019) -> (94.3571, -72.6177)
  line L481 (94.3571, -72.6177) -> (100, -75.8756)
  line L482 (100, -62.844) -> (94.3571, -66.1019)
  line L483 (-87.2143, -84.9899) -> (-87.2143, -78.4741)
  line L484 (-87.2143, -78.4741) -> (-92.8572, -75.2162)
  line L485 (-92.8572, -75.2162) -> (-98.5, -78.4741)
  line L486 (-98.5, -78.4741) -> (-98.5, -84.9899)
  line L487 (-92.8571, -88.2478) -> (-87.2143, -84.9899)
  line L488 (-98.5, -84.9899) -> (-92.8571, -88.2478)
  line L489 (-100, -100.6196) -> (-94.3571, -97.3617)
  line L490 (-94.3571, -97.3617) -> (-94.3572, -90.8459)
  line L491 (-94.3572, -90.8459) -> (-100, -87.588)
  line L492 (-72.9286, -84.9899) -> (-72.9286, -78.4741)
  line L493 (-72.9286, -78.4741) -> (-78.5714, -75.2162)
  line L494 (-78.5714, -75.2162) -> (-84.2143, -78.4741)
  line L495 (-84.2143, -78.4741) -> (-84.2143, -84.9899)
  line L496 (-78.5714, -88.2478) -> (-72.9286, -84.9899)
  line L497 (-84.2143, -84.9899) -> (-78.5714, -88.2478)
  line L498 (-91.3571, -90.8459) -> (-91.3571, -97.3617)
  line L499 (-91.3571, -97.3617) -> (-85.7143, -100.6196)
  line L500 (-85.7143, -100.6196) -> (-80.0714, -97.3617)
  line L501 (-80.0714, -97.3617) -> (-80.0714, -90.8459)
  line L502 (-85.7143, -87.588) -> (-91.3571, -90.8459)
  line L503 (-80.0714, -90.8459) -> (-85.7143, -87.588)
  line L504 (-58.6429, -84.9899) -> (-58.6429, -78.4741)
  line L505 (-58.6429, -78.4741) -> (-64.2857, -75.2162)
  line L506 (-64.2857, -75.2162) -> (-69.9286, -78.4741)
  line L507 (-69.9286, -78.4741) -> (-69.9286, -84.9899)
  line L508 (-64.2857, -88.2478) -> (-58.6429, -84.9899)
  line L509 (-69.9286, -84.9899) -> (-64.2857, -88.2478)
  line L510 (-77.0714, -90.8459) -> (-77.0714, -97.3617)
  line L511 (-77.0714, -97.3617) -> (-71.4286, -100.6196)
  line L512 (-71.4286, -100.6196) -> (-65.7857, -97.3617)
  line L513 (-65.7857, -97.3617) -> (-65.7857, -90.8459)
  line L514 (-71.4286, -87.588) -> (-77.0714, -90.8459)
  line L515 (-65.7857, -90.8459) -> (-71.4286, -87.588)
  line L516 (-44.3572, -84.9899) -> (-44.3572, -78.4741)
  line L517 (-44.3572, -78.4741) -> (-50, -75.2162)
  line L518 (-50, -75.2162) -> (-55.6429, -78.4741)
  line L519 (-55.6429, -78.4741) -> (-55.6429, -84.9899)
  line L520 (-50, -88.2478) -> (-44.3572, -84.9899)
  line L521 (-55.6429, -84.9899) -> (-50, -88.2478)
  line L522 (-62.7857, -90.8459) -> (-62.7857, -97.3617)
  line L523 (-62.7857, -97.3617) -> (-57.1429, -100.6196)
  line L524 (-57.1429, -100.6196) -> (-51.5, -97.3617)
  line L525 (-51.5, -97.3617) -> (-51.5, -90.8459)
  line L526 (-57.1429, -87.588) -> (-62.7857, -90.8459)
  line L527 (-51.5, -90.8459) -> (-57.1429, -87.588)
  line L528 (-30.0714, -84.9899) -> (-30.0714, -78.4741)
  line L529 (-30.0714, -78.4741) -> (-35.7143, -75.2162)
  line L530 (-35.7143, -75.2162) -> (-41.3571, -78.4741)
  line L531 (-41.3571, -78.4741) -> (-41.3571, -84.9899)
  line L532 (-35.7143, -88.2478) -> (-30.0714, -84.9899)
  line L533 (-41.3571, -84.9899) -> (-35.7143, -88.2478)
  line L534 (-48.5, -90.8459) -> (-48.5, -97.3617)
  line L535 (-48.5, -97.3617) -> (-42.8571, -100.6196)
  line L536 (-42.8571, -100.6196) -> (-37.2143, -97.3617)
  line L537 (-37.2143, -97.3617) -> (-37.2143, -90.8459)
  line L538 (-42.8571, -87.588) -> (-48.5, -90.8459)
  line L539 (-37.2143, -90.8459) -> (-42.8571, -87.588)
  line L540 (-15.7857, -84.9899) -> (-15.7857, -78.4741)
  line L541 (-15.7857, -78.4741) -> (-21.4286, -75.2162)
  line L542 (-21.4286, -75.2162) -> (-27.0714, -78.4741)
  line L543 (-27.0714, -78.4741) -> (-27.0714, -84.9899)
  line L544 (-21.4286, -88.2478) -> (-15.7857, -84.9899)
  line L545 (-34.2143, -90.8459) -> (-34.2143, -97.3617)
  line L546 (-34.2143, -97.3617) -> (-28.5714, -100.6196)
  line L547 (-28.5714, -100.6196) -> (-22.9286, -97.3617)
  line L548 (-22.9286, -97.3617) -> (-22.9286, -90.8459)
  line L549 (-28.5714, -87.588) -> (-34.2143, -90.8459)
  line L550 (-22.9286, -90.8459) -> (-28.5714, -87.588)
  line L551 (-1.5, -84.9899) -> (-1.5, -78.4741)
  line L552 (-1.5, -78.4741) -> (-7.1429, -75.2162)
  line L553 (-7.1429, -75.2162) -> (-12.7857, -78.4741)
  line L554 (-12.7857, -78.4741) -> (-12.7857, -84.9899)
  line L555 (-7.1429, -88.2478) -> (-1.5, -84.9899)
  line L556 (-12.7857, -84.9899) -> (-7.1429, -88.2478)
  line L557 (-19.9286, -90.8459) -> (-19.9286, -97.3617)
  line L558 (-19.9286, -97.3617) -> (-14.2857, -100.6196)
  line L559 (-14.2857, -100.6196) -> (-8.6429, -97.3617)
  line L560 (-8.6429, -97.3617) -> (-8.6429, -90.8459)
  line L561 (-14.2857, -87.588) -> (-19.9286, -90.8459)
  line L562 (-8.6429, -90.8459) -> (-14.2857, -87.588)
  line L563 (12.7854, -84.9897) -> (12.7854, -78.4739)
  line L564 (12.7854, -78.4739) -> (7.1428, -75.2162)
  line L565 (7.1428, -75.2162) -> (1.5, -78.4741)
  line L566 (1.5, -78.4741) -> (1.5, -84.9899)
  line L567 (1.5, -84.9899) -> (7.1424, -88.2475)
  line L568 (-5.6429, -90.8459) -> (-5.6429, -97.3617)
  line L569 (-5.6429, -97.3617) -> (0, -100.6196)
  line L570 (0, -100.6196) -> (5.6424, -97.3619)
  line L571 (-0.0003, -87.5881) -> (-5.6429, -90.8459)
  line L572 (5.6426, -90.846) -> (-0.0003, -87.5881)
  line L573 (27.0714, -84.9896) -> (27.0714, -78.4741)
  line L574 (27.0714, -78.4741) -> (21.4286, -75.2162)
  line L575 (21.4286, -75.2162) -> (15.7857, -78.4741)
  line L576 (15.7857, -78.4741) -> (15.7857, -84.9894)
  line L577 (21.4286, -88.2475) -> (27.0714, -84.9896)
  line L578 (8.6429, -90.8459) -> (8.6429, -97.3617)
  line L579 (8.6429, -97.3617) -> (14.2857, -100.6196)
  line L580 (14.2857, -100.6196) -> (19.9286, -97.3617)
  line L581 (19.9286, -97.3617) -> (19.9286, -90.8459)
  line L582 (14.2857, -87.588) -> (8.6429, -90.8459)
  line L583 (19.9286, -90.8459) -> (14.2857, -87.588)
  line L584 (41.3571, -84.9899) -> (41.3571, -78.4741)
  line L585 (41.3571, -78.4741) -> (35.7143, -75.2162)
  line L586 (35.7143, -75.2162) -> (30.0714, -78.4741)
  line L587 (30.0714, -78.4741) -> (30.0714, -84.9899)
  line L588 (35.7143, -88.2478) -> (41.3571, -84.9899)
  line L589 (30.0714, -84.9899) -> (35.7143, -88.2478)
  line L590 (22.9289, -97.3615) -> (28.5717, -100.6194)
  line L591 (28.5717, -100.6194) -> (34.2143, -97.3617)
  line L592 (34.2143, -97.3617) -> (34.2143, -90.8459)
  line L593 (28.5714, -87.588) -> (22.929, -90.8456)
  line L594 (34.2143, -90.8459) -> (28.5714, -87.588)
  line L595 (55.6428, -84.9899) -> (55.6428, -78.4741)
  line L596 (55.6428, -78.4741) -> (50, -75.2162)
  line L597 (50, -75.2162) -> (44.3571, -78.4741)
  line L598 (44.3571, -78.4741) -> (44.3571, -84.9899)
  line L599 (50, -88.2478) -> (55.6428, -84.9899)
  line L600 (44.3571, -84.9899) -> (50, -88.2478)
  line L601 (37.2143, -90.8459) -> (37.2143, -97.3617)
  line L602 (37.2143, -97.3617) -> (42.8571, -100.6196)
  line L603 (42.8571, -100.6196) -> (48.5, -97.3617)
  line L604 (48.5, -97.3617) -> (48.5, -90.8459)
  line L605 (42.8571, -87.588) -> (37.2143, -90.8459)
  line L606 (48.5, -90.8459) -> (42.8571, -87.588)
  line L607 (69.9286, -84.9899) -> (69.9286, -78.4741)
  line L608 (69.9286, -78.4741) -> (64.2857, -75.2162)
  line L609 (64.2857, -75.2162) -> (58.6429, -78.4741)
  line L610 (58.6429, -78.4741) -> (58.6429, -84.9899)
  line L611 (64.2857, -88.2478) -> (69.9286, -84.9899)
  line L612 (58.6429, -84.9899) -> (64.2857, -88.2478)
  line L613 (51.5, -90.8459) -> (51.5, -97.3617)
  line L614 (51.5, -97.3617) -> (57.1429, -100.6196)
  line L615 (57.1429, -100.6196) -> (62.7857, -97.3617)
  line L616 (62.7857, -97.3617) -> (62.7857, -90.8459)
  line L617 (57.1429, -87.588) -> (51.5, -90.8459)
  line L618 (62.7857, -90.8459) -> (57.1429, -87.588)
  line L619 (84.2143, -84.9899) -> (84.2143, -78.4741)
  line L620 (84.2143, -78.4741) -> (78.5714, -75.2162)
  line L621 (78.5714, -75.2162) -> (72.9286, -78.4741)
  line L622 (72.9286, -78.4741) -> (72.9286, -84.9899)
  line L623 (78.5714, -88.2478) -> (84.2143, -84.9899)
  line L624 (72.9286, -84.9899) -> (78.5714, -88.2478)
  line L625 (65.7857, -90.8459) -> (65.7857, -97.3617)
  line L626 (65.7857, -97.3617) -> (71.429, -100.6198)
  line L627 (77.0718, -97.3619) -> (77.0718, -90.8461)
  line L628 (71.4286, -87.588) -> (65.7857, -90.8459)
  line L629 (77.0718, -90.8461) -> (71.4286, -87.588)
  line L630 (98.5, -84.9899) -> (98.5, -78.4741)
  line L631 (98.5, -78.4741) -> (92.8571, -75.2162)
  line L632 (92.8571, -75.2162) -> (87.2143, -78.4741)
  line L633 (87.2143, -78.4741) -> (87.2143, -84.9899)
  line L634 (92.8571, -88.2478) -> (98.5, -84.9899)
  line L635 (87.2143, -84.9899) -> (92.8571, -88.2478)
  line L636 (80.0714, -90.8459) -> (80.0714, -97.3621)
  line L637 (85.7143, -100.62) -> (91.3571, -97.3621)
  line L638 (91.3571, -97.3621) -> (91.3571, -90.8459)
  line L639 (85.7143, -87.588) -> (80.0714, -90.8459)
  line L640 (91.3571, -90.8459) -> (85.7143, -87.588)
  line L641 (94.3571, -90.8459) -> (94.3571, -97.3617)
  line L642 (94.3571, -97.3617) -> (100, -100.6196)
  line L643 (100, -87.588) -> (94.3571, -90.8459)
  line L644 (-87.2143, -109.7339) -> (-87.2143, -103.2181)
  line L645 (-87.2143, -103.2181) -> (-92.8572, -99.9602)
  line L646 (-92.8572, -99.9602) -> (-98.5, -103.2181)
  line L647 (-98.5, -103.2181) -> (-98.5, -109.7339)
  line L648 (-92.8571, -112.9918) -> (-87.2143, -109.7339)
  line L649 (-98.5, -109.7339) -> (-92.8571, -112.9918)
  line L650 (-100, -125.3636) -> (-94.3571, -122.1057)
  line L651 (-94.3571, -122.1057) -> (-94.3572, -115.5899)
  line L652 (-94.3572, -115.5899) -> (-100, -112.332)
  line L653 (-72.9286, -109.7339) -> (-72.9286, -103.2181)
  line L654 (-72.9286, -103.2181) -> (-78.5714, -99.9602)
  line L655 (-78.5714, -99.9602) -> (-84.2143, -103.2181)
  line L656 (-84.2143, -103.2181) -> (-84.2143, -109.7339)
  line L657 (-78.5714, -112.9918) -> (-72.9286, -109.7339)
  line L658 (-84.2143, -109.7339) -> (-78.5714, -112.9918)
  line L659 (-91.3571, -115.5899) -> (-91.3571, -122.1057)
  line L660 (-91.3571, -122.1057) -> (-85.7143, -125.3636)
  line L661 (-85.7143, -125.3636) -> (-80.0714, -122.1057)
  line L662 (-80.0714, -122.1057) -> (-80.0714, -115.5899)
  line L663 (-85.7143, -112.332) -> (-91.3571, -115.5899)
  line L664 (-80.0714, -115.5899) -> (-85.7143, -112.332)
  line L665 (-58.6429, -109.7339) -> (-58.6429, -103.2181)
  line L666 (-58.6429, -103.2181) -> (-64.2857, -99.9602)
  line L667 (-64.2857, -99.9602) -> (-69.9286, -103.2181)
  line L668 (-69.9286, -103.2181) -> (-69.9286, -109.7339)
  line L669 (-64.2857, -112.9918) -> (-58.6429, -109.7339)
  line L670 (-69.9286, -109.7339) -> (-64.2857, -112.9918)
  line L671 (-77.0714, -115.5899) -> (-77.0714, -122.1057)
  line L672 (-77.0714, -122.1057) -> (-71.4286, -125.3636)
  line L673 (-71.4286, -125.3636) -> (-65.7857, -122.1057)
  line L674 (-65.7857, -122.1057) -> (-65.7857, -115.5899)
  line L675 (-71.4286, -112.332) -> (-77.0714, -115.5899)
  line L676 (-65.7857, -115.5899) -> (-71.4286, -112.332)
  line L677 (-44.3572, -109.7339) -> (-44.3572, -103.2181)
  line L678 (-44.3572, -103.2181) -> (-50, -99.9602)
  line L679 (-50, -99.9602) -> (-55.6429, -103.2181)
  line L680 (-55.6429, -103.2181) -> (-55.6429, -109.7339)
  line L681 (-50, -112.9918) -> (-44.3572, -109.7339)
  line L682 (-55.6429, -109.7339) -> (-50, -112.9918)
  line L683 (-62.7857, -115.5899) -> (-62.7857, -122.1057)
  line L684 (-62.7857, -122.1057) -> (-57.1429, -125.3636)
  line L685 (-57.1429, -125.3636) -> (-51.5, -122.1057)
  line L686 (-51.5, -122.1057) -> (-51.5, -115.5899)
  line L687 (-57.1429, -112.332) -> (-62.7857, -115.5899)
  line L688 (-51.5, -115.5899) -> (-57.1429, -112.332)
  line L689 (-30.0714, -109.7339) -> (-30.0714, -103.2181)
  line L690 (-30.0714, -103.2181) -> (-35.7143, -99.9602)
  line L691 (-35.7143, -99.9602) -> (-41.3571, -103.2181)
  line L692 (-41.3571, -103.2181) -> (-41.3571, -109.7339)
  line L693 (-35.7143, -112.9918) -> (-30.0714, -109.7339)
  line L694 (-41.3571, -109.7339) -> (-35.7143, -112.9918)
  line L695 (-48.5, -115.5899) -> (-48.5, -122.1057)
  line L696 (-48.5, -122.1057) -> (-42.8571, -125.3636)
  line L697 (-42.8571, -125.3636) -> (-37.2143, -122.1057)
  line L698 (-37.2143, -122.1057) -> (-37.2143, -115.5899)
  line L699 (-42.8571, -112.332) -> (-48.5, -115.5899)
  line L700 (-37.2143, -115.5899) -> (-42.8571, -112.332)
  line L701 (-15.7857, -109.7339) -> (-15.7857, -103.2181)
  line L702 (-15.7857, -103.2181) -> (-21.4286, -99.9602)
  line L703 (-21.4286, -99.9602) -> (-27.0714, -103.2181)
  line L704 (-27.0714, -103.2181) -> (-27.0714, -109.7339)
  line L705 (-21.4286, -112.9918) -> (-15.7857, -109.7339)
  line L706 (-27.0714, -109.7339) -> (-21.4286, -112.9918)
  line L707 (-34.2143, -115.5899) -> (-34.2143, -122.1057)
  line L708 (-34.2143, -122.1057) -> (-28.5714, -125.3636)
  line L709 (-28.5714, -125.3636) -> (-22.9286, -122.1057)
  line L710 (-22.9286, -122.1057) -> (-22.9286, -115.5899)
  line L711 (-28.5714, -112.332) -> (-34.2143, -115.5899)
  line L712 (-22.9286, -115.5899) -> (-28.5714, -112.332)
  line L713 (-1.5, -109.7339) -> (-1.5, -103.2181)
  line L714 (-1.5, -103.2181) -> (-7.1429, -99.9602)
  line L715 (-7.1429, -99.9602) -> (-12.7857, -103.2181)
  line L716 (-12.7857, -103.2181) -> (-12.7857, -109.7339)
  line L717 (-7.1429, -112.9918) -> (-1.5, -109.7339)
  line L718 (-12.7857, -109.7339) -> (-7.1429, -112.9918)
  line L719 (-19.9286, -115.5899) -> (-19.9286, -122.1057)
  line L720 (-19.9286, -122.1057) -> (-14.2853, -125.3638)
  line L721 (-8.6425, -122.1059) -> (-8.6425, -115.5901)
  line L722 (-14.2857, -112.332) -> (-19.9286, -115.5899)
  line L723 (-8.6425, -115.5901) -> (-14.2857, -112.332)
  line L724 (12.7857, -109.7339) -> (12.7857, -103.2182)
  line L725 (7.1428, -99.9601) -> (1.5, -103.218)
  line L726 (1.5, -103.218) -> (1.5, -109.7339)
  line L727 (7.1428, -112.9918) -> (12.7857, -109.7339)
  line L728 (1.5, -109.7339) -> (7.1428, -112.9918)
  line L729 (-5.6429, -115.5899) -> (-5.6429, -122.1061)
  line L730 (0, -125.364) -> (5.6428, -122.1061)
  line L731 (5.6428, -122.1061) -> (5.6428, -115.5899)
  line L732 (0, -112.332) -> (-5.6429, -115.5899)
  line L733 (5.6428, -115.5899) -> (0, -112.332)
  line L734 (27.0714, -109.7339) -> (27.0714, -103.2182)
  line L735 (27.0714, -103.2182) -> (21.4286, -99.9603)
  line L736 (15.7857, -103.218) -> (15.7857, -109.7339)
  line L737 (21.4286, -112.9918) -> (27.0714, -109.7339)
  line L738 (15.7857, -109.7339) -> (21.4286, -112.9918)
  line L739 (8.6429, -115.5899) -> (8.6429, -122.1057)
  line L740 (8.6429, -122.1057) -> (14.2857, -125.3636)
  line L741 (14.2857, -125.3636) -> (19.9286, -122.1057)
  line L742 (19.9286, -122.1057) -> (19.9286, -115.5899)
  line L743 (14.2857, -112.332) -> (8.6429, -115.5899)
  line L744 (19.9286, -115.5899) -> (14.2857, -112.332)
  line L745 (41.3571, -109.7339) -> (41.3571, -103.2181)
  line L746 (41.3571, -103.2181) -> (35.7143, -99.9602)
  line L747 (35.7143, -99.9602) -> (30.0714, -103.2181)
  line L748 (30.0714, -103.2181) -> (30.0714, -109.7339)
  line L749 (35.7143, -112.9918) -> (41.3571, -109.7339)
  line L750 (30.0714, -109.7339) -> (35.7143, -112.9918)
  line L751 (22.9286, -115.5899) -> (22.9286, -122.1057)
  line L752 (22.9286, -122.1057) -> (28.5714, -125.3636)
  line L753 (28.5714, -125.3636) -> (34.2143, -122.1057)
  line L754 (34.2143, -122.1057) -> (34.2143, -115.5899)
  line L755 (28.5714, -112.332) -> (22.9286, -115.5899)
  line L756 (34.2143, -115.5899) -> (28.5714, -112.332)
  line L757 (55.6428, -109.7339) -> (55.6428, -103.2181)
  line L758 (55.6428, -103.2181) -> (50, -99.9602)
  line L759 (50, -99.9602) -> (44.3571, -103.2181)
  line L760 (44.3571, -103.2181) -> (44.3571, -109.7339)
  line L761 (50, -112.9918) -> (55.6428, -109.7339)
  line L762 (44.3571, -109.7339) -> (50, -112.9918)
  line L763 (37.2143, -115.5899) -> (37.2143, -122.1057)
  line L764 (37.2143, -122.1057) -> (42.8571, -125.3636)
  line L765 (42.8571, -125.3636) -> (48.5, -122.1057)
  line L766 (48.5, -122.1057) -> (48.5, -115.5899)
  line L767 (42.8571, -112.332) -> (37.2143, -115.5899)
  line L768 (48.5, -115.5899) -> (42.8571, -112.332)
  line L769 (69.9286, -103.2181) -> (64.2857, -99.9602)
  line L770 (64.2857, -99.9602) -> (58.6429, -103.2181)
  line L771 (58.6429, -103.2181) -> (58.6429, -109.7339)
  line L772 (64.2857, -112.9918) -> (69.9286, -109.7339)
  line L773 (58.6429, -109.7339) -> (64.2857, -112.9918)
  line L774 (51.5, -115.5899) -> (51.5, -122.1057)
  line L775 (51.5, -122.1057) -> (57.1429, -125.3636)
  line L776 (57.1429, -125.3636) -> (62.7857, -122.1057)
  line L777 (62.7857, -122.1057) -> (62.7857, -115.5899)
  line L778 (57.1429, -112.332) -> (51.5, -115.5899)
  line L779 (62.7857, -115.5899) -> (57.1429, -112.332)
  line L780 (84.2143, -109.7339) -> (84.2143, -103.2181)
  line L781 (84.2143, -103.2181) -> (78.5714, -99.9602)
  line L782 (78.5714, -99.9602) -> (72.9286, -103.2181)
  line L783 (72.9286, -103.2181) -> (72.9286, -109.7339)
  line L784 (72.9286, -109.7339) -> (78.5714, -112.9918)
  line L785 (65.7857, -115.5899) -> (65.7857, -122.1057)
  line L786 (65.7857, -122.1057) -> (71.4281, -125.3633)
  line L787 (71.4281, -125.3633) -> (77.071, -122.1054)
  line L788 (71.4286, -112.332) -> (65.7857, -115.5899)
  line L789 (98.5, -109.7336) -> (98.5, -103.2181)
  line L790 (98.5, -103.2181) -> (92.8571, -99.9602)
  line L791 (92.8571, -99.9602) -> (87.2143, -103.2181)
  line L792 (92.8571, -112.9915) -> (98.5, -109.7336)
  line L793 (80.0714, -115.5899) -> (80.0714, -122.1057)
  line L794 (80.0714, -122.1057) -> (85.7143, -125.3636)
  line L795 (85.7143, -125.3636) -> (91.3571, -122.1057)
  line L796 (91.3571, -122.1057) -> (91.3571, -115.5899)
  line L797 (85.7143, -112.332) -> (80.0714, -115.5899)
  line L798 (91.3571, -115.5899) -> (85.7143, -112.332)
  line L799 (94.3574, -122.1137) -> (100, -125.3721)
  line L800 (100, -112.332) -> (94.3576, -115.5896)
  line L801 (-87.2143, -134.4779) -> (-87.2143, -127.9621)
  line L802 (-87.2143, -127.9621) -> (-92.8572, -124.7042)
  line L803 (-92.8572, -124.7042) -> (-98.5, -127.9621)
  line L804 (-98.5, -127.9621) -> (-98.5, -134.4779)
  line L805 (-92.8571, -137.7358) -> (-87.2143, -134.4779)
  line L806 (-98.5, -134.4779) -> (-92.8571, -137.7358)
  line L807 (-100, -150.1076) -> (-94.3571, -146.8497)
  line L808 (-94.3571, -146.8497) -> (-94.3572, -140.3339)
  line L809 (-94.3572, -140.3339) -> (-100, -137.076)
  line L810 (-72.9286, -134.4779) -> (-72.9286, -127.9621)
  line L811 (-72.9286, -127.9621) -> (-78.5714, -124.7042)
  line L812 (-78.5714, -124.7042) -> (-84.2143, -127.9621)
  line L813 (-84.2143, -127.9621) -> (-84.2143, -134.4779)
  line L814 (-78.5714, -137.7358) -> (-72.9286, -134.4779)
  line L815 (-84.2143, -134.4779) -> (-78.5714, -137.7358)
  line L816 (-91.3571, -140.3339) -> (-91.3571, -146.8497)
  line L817 (-91.3571, -146.8497) -> (-85.7143, -150.1076)
  line L818 (-85.7143, -150.1076) -> (-80.0714, -146.8497)
  line L819 (-80.0714, -146.8497) -> (-80.0714, -140.3339)
  line L820 (-85.7143, -137.076) -> (-91.3571, -140.3339)
  line L821 (-80.0714, -140.3339) -> (-85.7143, -137.076)
  line L822 (-58.6429, -134.4779) -> (-58.6429, -127.9621)
  line L823 (-58.6429, -127.9621) -> (-64.2857, -124.7042)
  line L824 (-64.2857, -124.7042) -> (-69.9286, -127.9621)
  line L825 (-69.9286, -127.9621) -> (-69.9286, -134.4779)
  line L826 (-64.2857, -137.7358) -> (-58.6429, -134.4779)
  line L827 (-69.9286, -134.4779) -> (-64.2857, -137.7358)
  line L828 (-77.0714, -140.3339) -> (-77.0714, -146.8497)
  line L829 (-77.0714, -146.8497) -> (-71.4286, -150.1076)
  line L830 (-71.4286, -150.1076) -> (-65.7857, -146.8497)
  line L831 (-65.7857, -146.8497) -> (-65.7857, -140.3339)
  line L832 (-71.4286, -137.076) -> (-77.0714, -140.3339)
  line L833 (-65.7857, -140.3339) -> (-71.4286, -137.076)
  line L834 (-44.3572, -134.4779) -> (-44.3572, -127.9621)
  line L835 (-44.3572, -127.9621) -> (-50, -124.7042)
  line L836 (-50, -124.7042) -> (-55.6429, -127.9621)
  line L837 (-55.6429, -127.9621) -> (-55.6429, -134.4779)
  line L838 (-50, -137.7358) -> (-44.3572, -134.4779)
  line L839 (-55.6429, -134.4779) -> (-50, -137.7358)
  line L840 (-62.7857, -140.3339) -> (-62.7857, -146.8497)
  line L841 (-62.7857, -146.8497) -> (-57.1429, -150.1076)
  line L842 (-57.1429, -150.1076) -> (-51.5, -146.8497)
  line L843 (-51.5, -146.8497) -> (-51.5, -140.3339)
  line L844 (-57.1429, -137.076) -> (-62.7857, -140.3339)
  line L845 (-51.5, -140.3339) -> (-57.1429, -137.076)
  line L846 (-30.0714, -134.4779) -> (-30.0714, -127.9621)
  line L847 (-30.0714, -127.9621) -> (-35.7143, -124.7042)
  line L848 (-35.7143, -124.7042) -> (-41.3571, -127.9621)
  line L849 (-41.3571, -127.9621) -> (-41.3571, -134.4779)
  line L850 (-35.7143, -137.7358) -> (-30.0714, -134.4779)
  line L851 (-41.3571, -134.4779) -> (-35.7143, -137.7358)
  line L852 (-48.5, -140.3339) -> (-48.5, -146.8497)
  line L853 (-48.5, -146.8497) -> (-45.9892, -148.2993)
  line L854 (-37.2143, -146.5) -> (-37.2143, -140.3339)
  line L855 (-42.8571, -137.076) -> (-48.5, -140.3339)
  line L856 (-37.2143, -140.3339) -> (-42.8571, -137.076)
  line L857 (-15.7857, -127.9621) -> (-21.4286, -124.7042)
  line L858 (-21.4286, -124.7042) -> (-27.0714, -127.9621)
  line L859 (-27.0714, -127.9621) -> (-27.0714, -134.4779)
  line L860 (-21.4286, -137.7358) -> (-15.7857, -134.4779)
  line L861 (-27.0714, -134.4779) -> (-21.4286, -137.7358)
  line L862 (-34.2143, -140.3339) -> (-34.2143, -146.5)
  line L863 (-22.9286, -146.5) -> (-22.9286, -140.3339)
  line L864 (-28.5714, -137.076) -> (-34.2143, -140.3339)
  line L865 (-22.9286, -140.3339) -> (-28.5714, -137.076)
  line L866 (-1.5, -134.4779) -> (-1.5, -127.9621)
  line L867 (-1.5, -127.9621) -> (-7.1429, -124.7042)
  line L868 (-7.1429, -124.7042) -> (-12.7857, -127.9621)
  line L869 (-12.7857, -127.9621) -> (-12.7857, -134.4779)
  line L870 (-7.1429, -137.7358) -> (-1.5, -134.4779)
  line L871 (-12.7857, -134.4779) -> (-7.1429, -137.7358)
  line L872 (-19.9286, -140.3339) -> (-19.9286, -146.5)
  line L873 (-8.6429, -146.5) -> (-8.6429, -140.3339)
  line L874 (-14.2857, -137.076) -> (-19.9286, -140.3339)
  line L875 (12.7857, -134.4779) -> (12.7857, -127.9621)
  line L876 (12.7857, -127.9621) -> (7.1428, -124.7042)
  line L877 (7.1428, -124.7042) -> (1.5, -127.9621)
  line L878 (7.1428, -137.7358) -> (12.7857, -134.4779)
  line L879 (1.5, -134.4779) -> (7.1428, -137.7358)
  line L880 (-5.6429, -140.3339) -> (-5.6429, -146.5)
  line L881 (5.6428, -146.5) -> (5.6428, -140.3339)
  line L882 (5.6428, -140.3339) -> (0, -137.076)
  line L883 (27.0714, -134.4779) -> (27.0714, -127.9621)
  line L884 (27.0714, -127.9621) -> (21.4286, -124.7042)